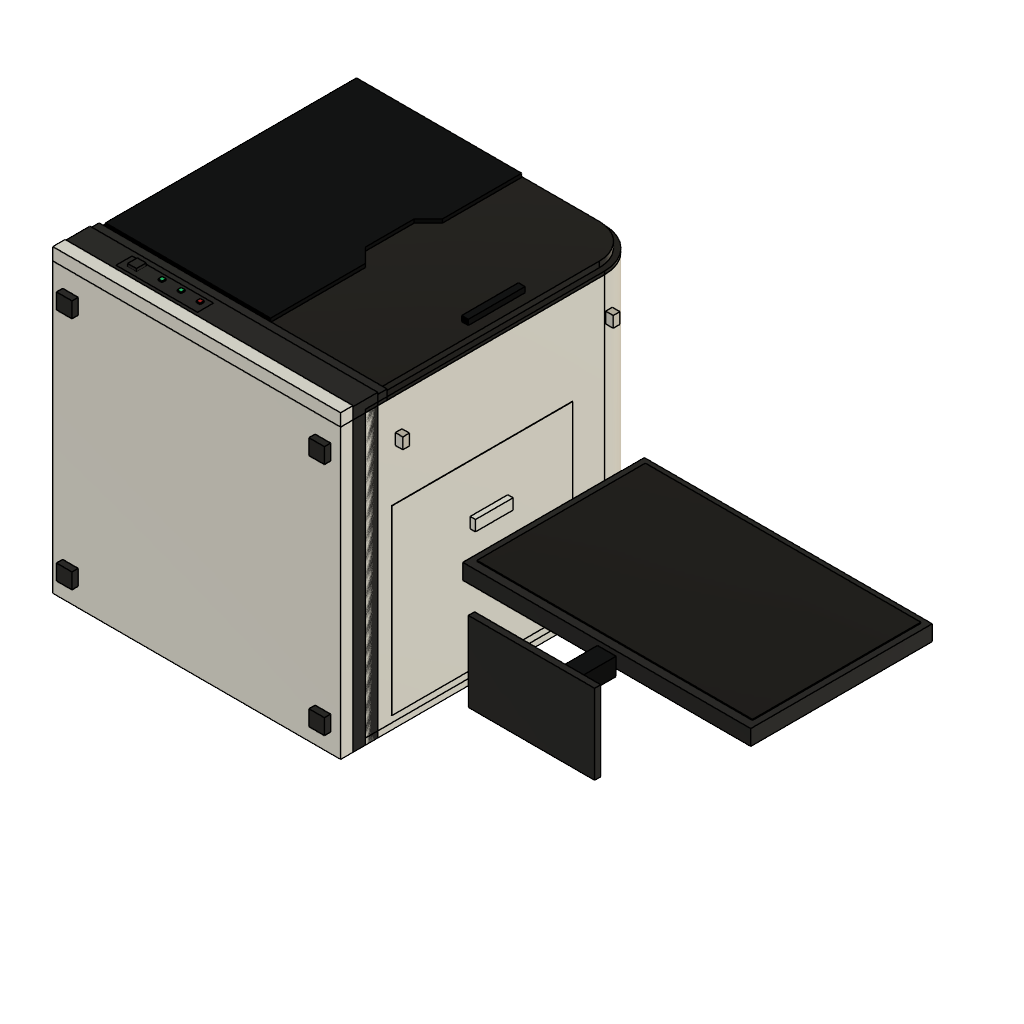
S60-before-branding (Autodesk Fusion 360 design; units mm, degrees)
Autodesk Fusion 360 part; units mm, degrees
(part 1 of 3)
ref_plane "WorkPlane1" through (0, 0, -280) normal (0, 0, 1) x (1, 0, 0) in component "cassette_bays | Three vertical cassette bays | DEPTH PROVISIONAL"
sketch "bay_back profile" plane through (0, 0, -280) normal (0, 0, 1) x (1, 0, 0) in component "cassette_bays | Three vertical cassette bays | DEPTH PROVISIONAL"
  line L0 (142, 117.5) -> (268, 117.5)
  line L1 (268, 117.5) -> (268, 592.5)
  line L2 (268, 592.5) -> (142, 592.5)
  line L3 (142, 592.5) -> (142, 117.5)
extrude "bay_back solid extrusion" add sketch "bay_back profile" along normal blind 9 makes body 1 in component "cassette_bays | Three vertical cassette bays | DEPTH PROVISIONAL"
ref_plane "WorkPlane2" through (0, 0, -275.5) normal (0, 0, 1) x (1, 0, 0) in component "cassette_bays | Three vertical cassette bays | DEPTH PROVISIONAL"
sketch "side_frame profile" plane through (0, 0, -275.5) normal (0, 0, 1) x (1, 0, 0) in component "cassette_bays | Three vertical cassette bays | DEPTH PROVISIONAL"
  line L0 (140, 118) -> (150, 118)
  line L1 (150, 118) -> (150, 592)
  line L2 (150, 592) -> (140, 592)
  line L3 (140, 592) -> (140, 118)
  line L4 (260, 118) -> (270, 118)
  line L5 (270, 118) -> (270, 592)
  line L6 (270, 592) -> (260, 592)
  line L7 (260, 592) -> (260, 118)
extrude "side_frame solid extrusion" add sketch "side_frame profile" along normal blind 108 separate body makes body 2 at (140, 434, -239.5) makes body 3 at (260, 434, -239.5) in component "cassette_bays | Three vertical cassette bays | DEPTH PROVISIONAL"
ref_plane "WorkPlane3" through (0, 0, -275.5) normal (0, 0, 1) x (1, 0, 0) in component "cassette_bays | Three vertical cassette bays | DEPTH PROVISIONAL"
sketch "cross_frame profile" plane through (0, 0, -275.5) normal (0, 0, 1) x (1, 0, 0) in component "cassette_bays | Three vertical cassette bays | DEPTH PROVISIONAL"
  line L0 (140, 116) -> (270, 116)
  line L1 (270, 116) -> (270, 126)
  line L2 (270, 126) -> (140, 126)
  line L3 (140, 126) -> (140, 116)
  line L4 (140, 275) -> (270, 275)
  line L5 (270, 275) -> (270, 285)
  line L6 (270, 285) -> (140, 285)
  line L7 (140, 285) -> (140, 275)
  line L8 (140, 425) -> (270, 425)
  line L9 (270, 425) -> (270, 435)
  line L10 (270, 435) -> (140, 435)
  line L11 (140, 435) -> (140, 425)
  line L12 (140, 584) -> (270, 584)
  line L13 (270, 584) -> (270, 594)
  line L14 (270, 594) -> (140, 594)
  line L15 (140, 594) -> (140, 584)
extrude "cross_frame solid extrusion" add sketch "cross_frame profile" along normal blind 108 separate body makes body 4 at (226.6667, 435, -239.5) makes body 5 at (226.6667, 285, -239.5) makes body 6 at (226.6667, 126, -239.5) makes body 7 at (226.6667, 594, -239.5) in component "cassette_bays | Three vertical cassette bays | DEPTH PROVISIONAL"
ref_plane "WorkPlane4" through (0, 0, -165.5) normal (0, 0, 1) x (1, 0, 0) in component "cassette_bays | Three vertical cassette bays | DEPTH PROVISIONAL"
sketch "seat_led_0 profile" plane through (0, 0, -165.5) normal (0, 0, 1) x (1, 0, 0) in component "cassette_bays | Three vertical cassette bays | DEPTH PROVISIONAL"
  line L0 (144, 264) -> (150, 264)
  line L1 (150, 264) -> (150, 270)
  line L2 (150, 270) -> (144, 270)
  line L3 (144, 270) -> (144, 264)
extrude "seat_led_0 solid extrusion" add sketch "seat_led_0 profile" along normal blind 4 separate body makes body 8 in component "cassette_bays | Three vertical cassette bays | DEPTH PROVISIONAL"
ref_plane "WorkPlane5" through (0, 0, -165.5) normal (0, 0, 1) x (1, 0, 0) in component "cassette_bays | Three vertical cassette bays | DEPTH PROVISIONAL"
sketch "seat_led_1 profile" plane through (0, 0, -165.5) normal (0, 0, 1) x (1, 0, 0) in component "cassette_bays | Three vertical cassette bays | DEPTH PROVISIONAL"
  line L0 (144, 414) -> (150, 414)
  line L1 (150, 414) -> (150, 420)
  line L2 (150, 420) -> (144, 420)
  line L3 (144, 420) -> (144, 414)
extrude "seat_led_1 solid extrusion" add sketch "seat_led_1 profile" along normal blind 4 separate body makes body 9 in component "cassette_bays | Three vertical cassette bays | DEPTH PROVISIONAL"
ref_plane "WorkPlane6" through (0, 0, -165.5) normal (0, 0, 1) x (1, 0, 0) in component "cassette_bays | Three vertical cassette bays | DEPTH PROVISIONAL"
sketch "seat_led_2 profile" plane through (0, 0, -165.5) normal (0, 0, 1) x (1, 0, 0) in component "cassette_bays | Three vertical cassette bays | DEPTH PROVISIONAL"
  line L0 (144, 564) -> (150, 564)
  line L1 (150, 564) -> (150, 570)
  line L2 (150, 570) -> (144, 570)
  line L3 (144, 570) -> (144, 564)
extrude "seat_led_2 solid extrusion" add sketch "seat_led_2 profile" along normal blind 4 separate body makes body 10 in component "cassette_bays | Three vertical cassette bays | DEPTH PROVISIONAL"
ref_plane "WorkPlane1" through (0, 0, -269.5) normal (0, 0, 1) x (1, 0, 0) in component "cassette_0 | Bottom cassette | DEPTH PROVISIONAL"
sketch "rack_base profile" plane through (0, 0, -269.5) normal (0, 0, 1) x (1, 0, 0) in component "cassette_0 | Bottom cassette | DEPTH PROVISIONAL"
  line L0 (165, 139) -> (245, 139)
  line L1 (245, 139) -> (245, 145)
  line L2 (245, 145) -> (165, 145)
  line L3 (165, 145) -> (165, 139)
extrude "rack_base solid extrusion" add sketch "rack_base profile" along normal blind 96 separate body makes body 11 in component "cassette_0 | Bottom cassette | DEPTH PROVISIONAL"
ref_plane "WorkPlane2" through (0, 0, -269.5) normal (0, 0, 1) x (1, 0, 0) in component "cassette_0 | Bottom cassette | DEPTH PROVISIONAL"
sketch "rack_top profile" plane through (0, 0, -269.5) normal (0, 0, 1) x (1, 0, 0) in component "cassette_0 | Bottom cassette | DEPTH PROVISIONAL"
  line L0 (165, 265.5) -> (245, 265.5)
  line L1 (245, 265.5) -> (245, 270.5)
  line L2 (245, 270.5) -> (165, 270.5)
  line L3 (165, 270.5) -> (165, 265.5)
extrude "rack_top solid extrusion" add sketch "rack_top profile" along normal blind 96 separate body makes body 12 in component "cassette_0 | Bottom cassette | DEPTH PROVISIONAL"
ref_plane "WorkPlane3" through (0, 0, -269.5) normal (0, 0, 1) x (1, 0, 0) in component "cassette_0 | Bottom cassette | DEPTH PROVISIONAL"
sketch "outer_guide profile" plane through (0, 0, -269.5) normal (0, 0, 1) x (1, 0, 0) in component "cassette_0 | Bottom cassette | DEPTH PROVISIONAL"
  line L0 (165, 143.5) -> (169, 143.5)
  line L1 (169, 143.5) -> (169, 266.5)
  line L2 (169, 266.5) -> (165, 266.5)
  line L3 (165, 266.5) -> (165, 143.5)
  line L4 (241, 143.5) -> (245, 143.5)
  line L5 (245, 143.5) -> (245, 266.5)
  line L6 (245, 266.5) -> (241, 266.5)
  line L7 (241, 266.5) -> (241, 143.5)
extrude "outer_guide solid extrusion" add sketch "outer_guide profile" along normal blind 96 separate body makes body 13 at (165, 225.5, -237.5) makes body 14 at (241, 225.5, -237.5) in component "cassette_0 | Bottom cassette | DEPTH PROVISIONAL"
ref_plane "WorkPlane4" through (0, 0, -177.5) normal (0, 0, 1) x (1, 0, 0) in component "cassette_0 | Bottom cassette | DEPTH PROVISIONAL"
sketch "rear_rib_PHOTO_ESTIMATE profile" plane through (0, 0, -177.5) normal (0, 0, 1) x (1, 0, 0) in component "cassette_0 | Bottom cassette | DEPTH PROVISIONAL"
  line L0 (168.5, 144) -> (175.5, 144)
  line L1 (175.5, 144) -> (175.5, 266)
  line L2 (175.5, 266) -> (168.5, 266)
  line L3 (168.5, 266) -> (168.5, 144)
  line L4 (201.5, 144) -> (208.5, 144)
  line L5 (208.5, 144) -> (208.5, 266)
  line L6 (208.5, 266) -> (201.5, 266)
  line L7 (201.5, 266) -> (201.5, 144)
  line L8 (234.5, 144) -> (241.5, 144)
  line L9 (241.5, 144) -> (241.5, 266)
  line L10 (241.5, 266) -> (234.5, 266)
  line L11 (234.5, 266) -> (234.5, 144)
extrude "rear_rib_PHOTO_ESTIMATE solid extrusion" add sketch "rear_rib_PHOTO_ESTIMATE profile" along normal blind 4 separate body makes body 15 at (170.8333, 184.6667, -177.5) makes body 16 at (203.8333, 225.3333, -177.5) makes body 17 at (236.8333, 184.6667, -177.5) in component "cassette_0 | Bottom cassette | DEPTH PROVISIONAL"
ref_plane "WorkPlane5" through (0, 0, -234) normal (0, 0, 1) x (1, 0, 0) in component "cassette_0 | Bottom cassette | DEPTH PROVISIONAL"
sketch "magnetic_base profile" plane through (0, 0, -234) normal (0, 0, 1) x (1, 0, 0) in component "cassette_0 | Bottom cassette | DEPTH PROVISIONAL"
  line L0 (191, 136.5) -> (219, 136.5)
  line L1 (219, 136.5) -> (219, 139.5)
  line L2 (219, 139.5) -> (191, 139.5)
  line L3 (191, 139.5) -> (191, 136.5)
extrude "magnetic_base solid extrusion" add sketch "magnetic_base profile" along normal blind 25 separate body makes body 18 in component "cassette_0 | Bottom cassette | DEPTH PROVISIONAL"
ref_plane "WorkPlane6" through (0, 0, -269.5) normal (0, 0, 1) x (1, 0, 0) in component "cassette_0 | Bottom cassette | DEPTH PROVISIONAL"
sketch "center_divider profile" plane through (0, 0, -269.5) normal (0, 0, 1) x (1, 0, 0) in component "cassette_0 | Bottom cassette | DEPTH PROVISIONAL"
  line L0 (203, 144) -> (207, 144)
  line L1 (207, 144) -> (207, 266)
  line L2 (207, 266) -> (203, 266)
  line L3 (203, 266) -> (203, 144)
extrude "center_divider solid extrusion" add sketch "center_divider profile" along normal blind 96 separate body makes body 19 in component "cassette_0 | Bottom cassette | DEPTH PROVISIONAL"
ref_plane "WorkPlane7" through (0, 0, -259.5) normal (0, 0, 1) x (1, 0, 0) in component "cassette_0 | Bottom cassette | DEPTH PROVISIONAL"
sketch "slide_glass profile" plane through (0, 0, -259.5) normal (0, 0, 1) x (1, 0, 0) in component "cassette_0 | Bottom cassette | DEPTH PROVISIONAL"
  line L0 (175, 253.5) -> (201, 253.5)
  line L1 (201, 253.5) -> (201, 254.5)
  line L2 (201, 254.5) -> (175, 254.5)
  line L3 (175, 254.5) -> (175, 253.5)
  line L4 (175, 243) -> (201, 243)
  line L5 (201, 243) -> (201, 244)
  line L6 (201, 244) -> (175, 244)
  line L7 (175, 244) -> (175, 243)
  line L8 (175, 232.5) -> (201, 232.5)
  line L9 (201, 232.5) -> (201, 233.5)
  line L10 (201, 233.5) -> (175, 233.5)
  line L11 (175, 233.5) -> (175, 232.5)
  line L12 (175, 222) -> (201, 222)
  line L13 (201, 222) -> (201, 223)
  line L14 (201, 223) -> (175, 223)
  line L15 (175, 223) -> (175, 222)
  line L16 (175, 211.5) -> (201, 211.5)
  line L17 (201, 211.5) -> (201, 212.5)
  line L18 (201, 212.5) -> (175, 212.5)
  line L19 (175, 212.5) -> (175, 211.5)
  line L20 (175, 201) -> (201, 201)
  line L21 (201, 201) -> (201, 202)
  line L22 (201, 202) -> (175, 202)
  line L23 (175, 202) -> (175, 201)
  line L24 (175, 190.5) -> (201, 190.5)
  line L25 (201, 190.5) -> (201, 191.5)
  line L26 (201, 191.5) -> (175, 191.5)
  line L27 (175, 191.5) -> (175, 190.5)
  line L28 (175, 180) -> (201, 180)
  line L29 (201, 180) -> (201, 181)
  line L30 (201, 181) -> (175, 181)
  line L31 (175, 181) -> (175, 180)
  line L32 (175, 169.5) -> (201, 169.5)
  line L33 (201, 169.5) -> (201, 170.5)
  line L34 (201, 170.5) -> (175, 170.5)
  line L35 (175, 170.5) -> (175, 169.5)
  line L36 (175, 159) -> (201, 159)
  line L37 (201, 159) -> (201, 160)
  line L38 (201, 160) -> (175, 160)
  line L39 (175, 160) -> (175, 159)
  line L40 (209, 253.5) -> (235, 253.5)
  line L41 (235, 253.5) -> (235, 254.5)
  line L42 (235, 254.5) -> (209, 254.5)
  line L43 (209, 254.5) -> (209, 253.5)
  line L44 (209, 243) -> (235, 243)
  line L45 (235, 243) -> (235, 244)
  line L46 (235, 244) -> (209, 244)
  line L47 (209, 244) -> (209, 243)
  line L48 (209, 232.5) -> (235, 232.5)
  line L49 (235, 232.5) -> (235, 233.5)
  line L50 (235, 233.5) -> (209, 233.5)
  line L51 (209, 233.5) -> (209, 232.5)
  line L52 (209, 222) -> (235, 222)
  line L53 (235, 222) -> (235, 223)
  line L54 (235, 223) -> (209, 223)
  line L55 (209, 223) -> (209, 222)
  line L56 (209, 211.5) -> (235, 211.5)
  line L57 (235, 211.5) -> (235, 212.5)
  line L58 (235, 212.5) -> (209, 212.5)
  line L59 (209, 212.5) -> (209, 211.5)
  line L60 (209, 201) -> (235, 201)
  line L61 (235, 201) -> (235, 202)
  line L62 (235, 202) -> (209, 202)
  line L63 (209, 202) -> (209, 201)
  line L64 (209, 190.5) -> (235, 190.5)
  line L65 (235, 190.5) -> (235, 191.5)
  line L66 (235, 191.5) -> (209, 191.5)
  line L67 (209, 191.5) -> (209, 190.5)
  line L68 (209, 180) -> (235, 180)
  line L69 (235, 180) -> (235, 181)
  line L70 (235, 181) -> (209, 181)
  line L71 (209, 181) -> (209, 180)
  line L72 (209, 169.5) -> (235, 169.5)
  line L73 (235, 169.5) -> (235, 170.5)
  line L74 (235, 170.5) -> (209, 170.5)
  line L75 (209, 170.5) -> (209, 169.5)
  line L76 (209, 159) -> (235, 159)
  line L77 (235, 159) -> (235, 160)
  line L78 (235, 160) -> (209, 160)
  line L79 (209, 160) -> (209, 159)
extrude "slide_glass solid extrusion" add sketch "slide_glass profile" along normal blind 76 separate body makes body 20 at (226.3333, 170.5, -234.1667) makes body 21 at (226.3333, 191.5, -234.1667) makes body 22 at (226.3333, 212.5, -234.1667) makes body 23 at (226.3333, 233.5, -234.1667) makes body 24 at (226.3333, 254.5, -234.1667) makes body 25 at (192.3333, 160, -234.1667) makes body 26 at (192.3333, 181, -234.1667) makes body 27 at (192.3333, 202, -234.1667) makes body 28 at (192.3333, 223, -234.1667) makes body 29 at (192.3333, 244, -234.1667) makes body 30 at (192.3333, 233.5, -234.1667) makes body 31 at (192.3333, 212.5, -234.1667) makes body 32 at (192.3333, 191.5, -234.1667) makes body 33 at (192.3333, 170.5, -234.1667) makes body 34 at (192.3333, 254.5, -234.1667) makes body 35 at (226.3333, 244, -234.1667) makes body 36 at (226.3333, 223, -234.1667) makes body 37 at (226.3333, 202, -234.1667) makes body 38 at (226.3333, 181, -234.1667) makes body 39 at (226.3333, 160, -234.1667) in component "cassette_0 | Bottom cassette | DEPTH PROVISIONAL"
ref_plane "WorkPlane8" through (0, 0, -263) normal (0, 0, 1) x (1, 0, 0) in component "cassette_0 | Bottom cassette | DEPTH PROVISIONAL"
sketch "slot_guide profile" plane through (0, 0, -263) normal (0, 0, 1) x (1, 0, 0) in component "cassette_0 | Bottom cassette | DEPTH PROVISIONAL"
  line L0 (173, 252) -> (175, 252)
  line L1 (175, 252) -> (175, 254)
  line L2 (175, 254) -> (173, 254)
  line L3 (173, 254) -> (173, 252)
  line L4 (201, 252) -> (203, 252)
  line L5 (203, 252) -> (203, 254)
  line L6 (203, 254) -> (201, 254)
  line L7 (201, 254) -> (201, 252)
  line L8 (173, 241.5) -> (175, 241.5)
  line L9 (175, 241.5) -> (175, 243.5)
  line L10 (175, 243.5) -> (173, 243.5)
  line L11 (173, 243.5) -> (173, 241.5)
  line L12 (201, 241.5) -> (203, 241.5)
  line L13 (203, 241.5) -> (203, 243.5)
  line L14 (203, 243.5) -> (201, 243.5)
  line L15 (201, 243.5) -> (201, 241.5)
  line L16 (173, 231) -> (175, 231)
  line L17 (175, 231) -> (175, 233)
  line L18 (175, 233) -> (173, 233)
  line L19 (173, 233) -> (173, 231)
  line L20 (201, 231) -> (203, 231)
  line L21 (203, 231) -> (203, 233)
  line L22 (203, 233) -> (201, 233)
  line L23 (201, 233) -> (201, 231)
  line L24 (173, 220.5) -> (175, 220.5)
  line L25 (175, 220.5) -> (175, 222.5)
  line L26 (175, 222.5) -> (173, 222.5)
  line L27 (173, 222.5) -> (173, 220.5)
  line L28 (201, 220.5) -> (203, 220.5)
  line L29 (203, 220.5) -> (203, 222.5)
  line L30 (203, 222.5) -> (201, 222.5)
  line L31 (201, 222.5) -> (201, 220.5)
  line L32 (173, 210) -> (175, 210)
  line L33 (175, 210) -> (175, 212)
  line L34 (175, 212) -> (173, 212)
  line L35 (173, 212) -> (173, 210)
  line L36 (201, 210) -> (203, 210)
  line L37 (203, 210) -> (203, 212)
  line L38 (203, 212) -> (201, 212)
  line L39 (201, 212) -> (201, 210)
  line L40 (173, 199.5) -> (175, 199.5)
  line L41 (175, 199.5) -> (175, 201.5)
  line L42 (175, 201.5) -> (173, 201.5)
  line L43 (173, 201.5) -> (173, 199.5)
  line L44 (201, 199.5) -> (203, 199.5)
  line L45 (203, 199.5) -> (203, 201.5)
  line L46 (203, 201.5) -> (201, 201.5)
  line L47 (201, 201.5) -> (201, 199.5)
  line L48 (173, 189) -> (175, 189)
  line L49 (175, 189) -> (175, 191)
  line L50 (175, 191) -> (173, 191)
  line L51 (173, 191) -> (173, 189)
  line L52 (201, 189) -> (203, 189)
  line L53 (203, 189) -> (203, 191)
  line L54 (203, 191) -> (201, 191)
  line L55 (201, 191) -> (201, 189)
  line L56 (173, 178.5) -> (175, 178.5)
  line L57 (175, 178.5) -> (175, 180.5)
  line L58 (175, 180.5) -> (173, 180.5)
  line L59 (173, 180.5) -> (173, 178.5)
  line L60 (201, 178.5) -> (203, 178.5)
  line L61 (203, 178.5) -> (203, 180.5)
  line L62 (203, 180.5) -> (201, 180.5)
  line L63 (201, 180.5) -> (201, 178.5)
  line L64 (173, 168) -> (175, 168)
  line L65 (175, 168) -> (175, 170)
  line L66 (175, 170) -> (173, 170)
  line L67 (173, 170) -> (173, 168)
  line L68 (201, 168) -> (203, 168)
  line L69 (203, 168) -> (203, 170)
  line L70 (203, 170) -> (201, 170)
  line L71 (201, 170) -> (201, 168)
  line L72 (173, 157.5) -> (175, 157.5)
  line L73 (175, 157.5) -> (175, 159.5)
  line L74 (175, 159.5) -> (173, 159.5)
  line L75 (173, 159.5) -> (173, 157.5)
  line L76 (201, 157.5) -> (203, 157.5)
  line L77 (203, 157.5) -> (203, 159.5)
  line L78 (203, 159.5) -> (201, 159.5)
  line L79 (201, 159.5) -> (201, 157.5)
  line L80 (207, 252) -> (209, 252)
  line L81 (209, 252) -> (209, 254)
  line L82 (209, 254) -> (207, 254)
  line L83 (207, 254) -> (207, 252)
  line L84 (235, 252) -> (237, 252)
  line L85 (237, 252) -> (237, 254)
  line L86 (237, 254) -> (235, 254)
  line L87 (235, 254) -> (235, 252)
  line L88 (207, 241.5) -> (209, 241.5)
  line L89 (209, 241.5) -> (209, 243.5)
  line L90 (209, 243.5) -> (207, 243.5)
  line L91 (207, 243.5) -> (207, 241.5)
  line L92 (235, 241.5) -> (237, 241.5)
  line L93 (237, 241.5) -> (237, 243.5)
  line L94 (237, 243.5) -> (235, 243.5)
  line L95 (235, 243.5) -> (235, 241.5)
  line L96 (207, 231) -> (209, 231)
  line L97 (209, 231) -> (209, 233)
  line L98 (209, 233) -> (207, 233)
  line L99 (207, 233) -> (207, 231)
  line L100 (235, 231) -> (237, 231)
  line L101 (237, 231) -> (237, 233)
  line L102 (237, 233) -> (235, 233)
  line L103 (235, 233) -> (235, 231)
  line L104 (207, 220.5) -> (209, 220.5)
  line L105 (209, 220.5) -> (209, 222.5)
  line L106 (209, 222.5) -> (207, 222.5)
  line L107 (207, 222.5) -> (207, 220.5)
  line L108 (235, 220.5) -> (237, 220.5)
  line L109 (237, 220.5) -> (237, 222.5)
  line L110 (237, 222.5) -> (235, 222.5)
  line L111 (235, 222.5) -> (235, 220.5)
  line L112 (207, 210) -> (209, 210)
  line L113 (209, 210) -> (209, 212)
  line L114 (209, 212) -> (207, 212)
  line L115 (207, 212) -> (207, 210)
  line L116 (235, 210) -> (237, 210)
  line L117 (237, 210) -> (237, 212)
  line L118 (237, 212) -> (235, 212)
  line L119 (235, 212) -> (235, 210)
  line L120 (207, 199.5) -> (209, 199.5)
  line L121 (209, 199.5) -> (209, 201.5)
  line L122 (209, 201.5) -> (207, 201.5)
  line L123 (207, 201.5) -> (207, 199.5)
  line L124 (235, 199.5) -> (237, 199.5)
  line L125 (237, 199.5) -> (237, 201.5)
  line L126 (237, 201.5) -> (235, 201.5)
  line L127 (235, 201.5) -> (235, 199.5)
  line L128 (207, 189) -> (209, 189)
  line L129 (209, 189) -> (209, 191)
  line L130 (209, 191) -> (207, 191)
  line L131 (207, 191) -> (207, 189)
  line L132 (235, 189) -> (237, 189)
  line L133 (237, 189) -> (237, 191)
  line L134 (237, 191) -> (235, 191)
  line L135 (235, 191) -> (235, 189)
  line L136 (207, 178.5) -> (209, 178.5)
  line L137 (209, 178.5) -> (209, 180.5)
  line L138 (209, 180.5) -> (207, 180.5)
  line L139 (207, 180.5) -> (207, 178.5)
  line L140 (235, 178.5) -> (237, 178.5)
  line L141 (237, 178.5) -> (237, 180.5)
  line L142 (237, 180.5) -> (235, 180.5)
  line L143 (235, 180.5) -> (235, 178.5)
  line L144 (207, 168) -> (209, 168)
  line L145 (209, 168) -> (209, 170)
  line L146 (209, 170) -> (207, 170)
  line L147 (207, 170) -> (207, 168)
  line L148 (235, 168) -> (237, 168)
  line L149 (237, 168) -> (237, 170)
  line L150 (237, 170) -> (235, 170)
  line L151 (235, 170) -> (235, 168)
  line L152 (207, 157.5) -> (209, 157.5)
  line L153 (209, 157.5) -> (209, 159.5)
  line L154 (209, 159.5) -> (207, 159.5)
  line L155 (207, 159.5) -> (207, 157.5)
  line L156 (235, 157.5) -> (237, 157.5)
  line L157 (237, 157.5) -> (237, 159.5)
  line L158 (237, 159.5) -> (235, 159.5)
  line L159 (235, 159.5) -> (235, 157.5)
extrude "slot_guide solid extrusion" add sketch "slot_guide profile" along normal blind 83 separate body makes body 40 at (207, 158.8333, -207.6667) makes body 41 at (207, 169.3333, -207.6667) makes body 42 at (207, 179.8333, -207.6667) makes body 43 at (209, 189.6667, -207.6667) makes body 44 at (207, 200.8333, -207.6667) makes body 45 at (207, 211.3333, -207.6667) makes body 46 at (207, 221.8333, -207.6667) makes body 47 at (207, 232.3333, -207.6667) makes body 48 at (209, 242.1667, -207.6667) makes body 49 at (207, 253.3333, -207.6667) makes body 50 at (201, 158.8333, -207.6667) makes body 51 at (201, 169.3333, -207.6667) makes body 52 at (201, 179.8333, -207.6667) makes body 53 at (203, 189.6667, -207.6667) makes body 54 at (201, 200.8333, -207.6667) makes body 55 at (201, 211.3333, -207.6667) makes body 56 at (201, 221.8333, -207.6667) makes body 57 at (201, 232.3333, -207.6667) makes body 58 at (203, 242.1667, -207.6667) makes body 59 at (201, 253.3333, -207.6667) makes body 60 at (175, 242.1667, -207.6667) makes body 61 at (173, 232.3333, -207.6667) makes body 62 at (173, 221.8333, -207.6667) makes body 63 at (173, 211.3333, -207.6667) makes body 64 at (173, 200.8333, -207.6667) makes body 65 at (175, 189.6667, -207.6667) makes body 66 at (173, 179.8333, -207.6667) makes body 67 at (173, 169.3333, -207.6667) makes body 68 at (173, 158.8333, -207.6667) makes body 69 at (173, 253.3333, -207.6667) makes body 70 at (235, 253.3333, -207.6667) makes body 71 at (237, 242.1667, -207.6667) makes body 72 at (235, 232.3333, -207.6667) makes body 73 at (235, 221.8333, -207.6667) makes body 74 at (235, 211.3333, -207.6667) makes body 75 at (235, 200.8333, -207.6667) makes body 76 at (237, 189.6667, -207.6667) makes body 77 at (235, 179.8333, -207.6667) makes body 78 at (235, 169.3333, -207.6667) makes body 79 at (235, 158.8333, -207.6667) in component "cassette_0 | Bottom cassette | DEPTH PROVISIONAL"
ref_plane "WorkPlane1" through (0, 0, -269.5) normal (0, 0, 1) x (1, 0, 0) in component "cassette_1 | Middle cassette | DEPTH PROVISIONAL"
sketch "rack_base profile (2)" plane through (0, 0, -269.5) normal (0, 0, 1) x (1, 0, 0) in component "cassette_1 | Middle cassette | DEPTH PROVISIONAL"
  line L0 (165, 289) -> (245, 289)
  line L1 (245, 289) -> (245, 295)
  line L2 (245, 295) -> (165, 295)
  line L3 (165, 295) -> (165, 289)
extrude "rack_base solid extrusion'" add sketch "rack_base profile (2)" along normal blind 96 separate body makes body 80 in component "cassette_1 | Middle cassette | DEPTH PROVISIONAL"
ref_plane "WorkPlane2" through (0, 0, -269.5) normal (0, 0, 1) x (1, 0, 0) in component "cassette_1 | Middle cassette | DEPTH PROVISIONAL"
sketch "rack_top profile (2)" plane through (0, 0, -269.5) normal (0, 0, 1) x (1, 0, 0) in component "cassette_1 | Middle cassette | DEPTH PROVISIONAL"
  line L0 (165, 415.5) -> (245, 415.5)
  line L1 (245, 415.5) -> (245, 420.5)
  line L2 (245, 420.5) -> (165, 420.5)
  line L3 (165, 420.5) -> (165, 415.5)
extrude "rack_top solid extrusion'" add sketch "rack_top profile (2)" along normal blind 96 separate body makes body 81 in component "cassette_1 | Middle cassette | DEPTH PROVISIONAL"
ref_plane "WorkPlane3" through (0, 0, -269.5) normal (0, 0, 1) x (1, 0, 0) in component "cassette_1 | Middle cassette | DEPTH PROVISIONAL"
sketch "outer_guide profile (2)" plane through (0, 0, -269.5) normal (0, 0, 1) x (1, 0, 0) in component "cassette_1 | Middle cassette | DEPTH PROVISIONAL"
  line L0 (165, 293.5) -> (169, 293.5)
  line L1 (169, 293.5) -> (169, 416.5)
  line L2 (169, 416.5) -> (165, 416.5)
  line L3 (165, 416.5) -> (165, 293.5)
  line L4 (241, 293.5) -> (245, 293.5)
  line L5 (245, 293.5) -> (245, 416.5)
  line L6 (245, 416.5) -> (241, 416.5)
  line L7 (241, 416.5) -> (241, 293.5)
extrude "outer_guide solid extrusion'" add sketch "outer_guide profile (2)" along normal blind 96 separate body makes body 82 at (165, 375.5, -237.5) makes body 83 at (241, 375.5, -237.5) in component "cassette_1 | Middle cassette | DEPTH PROVISIONAL"
ref_plane "WorkPlane4" through (0, 0, -177.5) normal (0, 0, 1) x (1, 0, 0) in component "cassette_1 | Middle cassette | DEPTH PROVISIONAL"
sketch "rear_rib_PHOTO_ESTIMATE profile (2)" plane through (0, 0, -177.5) normal (0, 0, 1) x (1, 0, 0) in component "cassette_1 | Middle cassette | DEPTH PROVISIONAL"
  line L0 (168.5, 294) -> (175.5, 294)
  line L1 (175.5, 294) -> (175.5, 416)
  line L2 (175.5, 416) -> (168.5, 416)
  line L3 (168.5, 416) -> (168.5, 294)
  line L4 (201.5, 294) -> (208.5, 294)
  line L5 (208.5, 294) -> (208.5, 416)
  line L6 (208.5, 416) -> (201.5, 416)
  line L7 (201.5, 416) -> (201.5, 294)
  line L8 (234.5, 294) -> (241.5, 294)
  line L9 (241.5, 294) -> (241.5, 416)
  line L10 (241.5, 416) -> (234.5, 416)
  line L11 (234.5, 416) -> (234.5, 294)
extrude "rear_rib_PHOTO_ESTIMATE solid extrusion'" add sketch "rear_rib_PHOTO_ESTIMATE profile (2)" along normal blind 4 separate body makes body 84 at (170.8333, 375.3333, -177.5) makes body 85 at (203.8333, 375.3333, -177.5) makes body 86 at (236.8333, 375.3333, -177.5) in component "cassette_1 | Middle cassette | DEPTH PROVISIONAL"
ref_plane "WorkPlane5" through (0, 0, -234) normal (0, 0, 1) x (1, 0, 0) in component "cassette_1 | Middle cassette | DEPTH PROVISIONAL"
sketch "magnetic_base profile (2)" plane through (0, 0, -234) normal (0, 0, 1) x (1, 0, 0) in component "cassette_1 | Middle cassette | DEPTH PROVISIONAL"
  line L0 (191, 286.5) -> (219, 286.5)
  line L1 (219, 286.5) -> (219, 289.5)
  line L2 (219, 289.5) -> (191, 289.5)
  line L3 (191, 289.5) -> (191, 286.5)
extrude "magnetic_base solid extrusion'" add sketch "magnetic_base profile (2)" along normal blind 25 separate body makes body 87 in component "cassette_1 | Middle cassette | DEPTH PROVISIONAL"
ref_plane "WorkPlane6" through (0, 0, -269.5) normal (0, 0, 1) x (1, 0, 0) in component "cassette_1 | Middle cassette | DEPTH PROVISIONAL"
sketch "center_divider profile (2)" plane through (0, 0, -269.5) normal (0, 0, 1) x (1, 0, 0) in component "cassette_1 | Middle cassette | DEPTH PROVISIONAL"
  line L0 (203, 294) -> (207, 294)
  line L1 (207, 294) -> (207, 416)
  line L2 (207, 416) -> (203, 416)
  line L3 (203, 416) -> (203, 294)
extrude "center_divider solid extrusion'" add sketch "center_divider profile (2)" along normal blind 96 separate body makes body 88 in component "cassette_1 | Middle cassette | DEPTH PROVISIONAL"
ref_plane "WorkPlane7" through (0, 0, -259.5) normal (0, 0, 1) x (1, 0, 0) in component "cassette_1 | Middle cassette | DEPTH PROVISIONAL"
sketch "slide_glass profile (2)" plane through (0, 0, -259.5) normal (0, 0, 1) x (1, 0, 0) in component "cassette_1 | Middle cassette | DEPTH PROVISIONAL"
  line L0 (175, 403.5) -> (201, 403.5)
  line L1 (201, 403.5) -> (201, 404.5)
  line L2 (201, 404.5) -> (175, 404.5)
  line L3 (175, 404.5) -> (175, 403.5)
  line L4 (175, 393) -> (201, 393)
  line L5 (201, 393) -> (201, 394)
  line L6 (201, 394) -> (175, 394)
  line L7 (175, 394) -> (175, 393)
  line L8 (175, 382.5) -> (201, 382.5)
  line L9 (201, 382.5) -> (201, 383.5)
  line L10 (201, 383.5) -> (175, 383.5)
  line L11 (175, 383.5) -> (175, 382.5)
  line L12 (175, 372) -> (201, 372)
  line L13 (201, 372) -> (201, 373)
  line L14 (201, 373) -> (175, 373)
  line L15 (175, 373) -> (175, 372)
  line L16 (175, 361.5) -> (201, 361.5)
  line L17 (201, 361.5) -> (201, 362.5)
  line L18 (201, 362.5) -> (175, 362.5)
  line L19 (175, 362.5) -> (175, 361.5)
  line L20 (175, 351) -> (201, 351)
  line L21 (201, 351) -> (201, 352)
  line L22 (201, 352) -> (175, 352)
  line L23 (175, 352) -> (175, 351)
  line L24 (175, 340.5) -> (201, 340.5)
  line L25 (201, 340.5) -> (201, 341.5)
  line L26 (201, 341.5) -> (175, 341.5)
  line L27 (175, 341.5) -> (175, 340.5)
  line L28 (175, 330) -> (201, 330)
  line L29 (201, 330) -> (201, 331)
  line L30 (201, 331) -> (175, 331)
  line L31 (175, 331) -> (175, 330)
  line L32 (175, 319.5) -> (201, 319.5)
  line L33 (201, 319.5) -> (201, 320.5)
  line L34 (201, 320.5) -> (175, 320.5)
  line L35 (175, 320.5) -> (175, 319.5)
  line L36 (175, 309) -> (201, 309)
  line L37 (201, 309) -> (201, 310)
  line L38 (201, 310) -> (175, 310)
  line L39 (175, 310) -> (175, 309)
  line L40 (209, 403.5) -> (235, 403.5)
  line L41 (235, 403.5) -> (235, 404.5)
  line L42 (235, 404.5) -> (209, 404.5)
  line L43 (209, 404.5) -> (209, 403.5)
  line L44 (209, 393) -> (235, 393)
  line L45 (235, 393) -> (235, 394)
  line L46 (235, 394) -> (209, 394)
  line L47 (209, 394) -> (209, 393)
  line L48 (209, 382.5) -> (235, 382.5)
  line L49 (235, 382.5) -> (235, 383.5)
  line L50 (235, 383.5) -> (209, 383.5)
  line L51 (209, 383.5) -> (209, 382.5)
  line L52 (209, 372) -> (235, 372)
  line L53 (235, 372) -> (235, 373)
  line L54 (235, 373) -> (209, 373)
  line L55 (209, 373) -> (209, 372)
  line L56 (209, 361.5) -> (235, 361.5)
  line L57 (235, 361.5) -> (235, 362.5)
  line L58 (235, 362.5) -> (209, 362.5)
  line L59 (209, 362.5) -> (209, 361.5)
  line L60 (209, 351) -> (235, 351)
  line L61 (235, 351) -> (235, 352)
  line L62 (235, 352) -> (209, 352)
  line L63 (209, 352) -> (209, 351)
  line L64 (209, 340.5) -> (235, 340.5)
  line L65 (235, 340.5) -> (235, 341.5)
  line L66 (235, 341.5) -> (209, 341.5)
  line L67 (209, 341.5) -> (209, 340.5)
  line L68 (209, 330) -> (235, 330)
  line L69 (235, 330) -> (235, 331)
  line L70 (235, 331) -> (209, 331)
  line L71 (209, 331) -> (209, 330)
  line L72 (209, 319.5) -> (235, 319.5)
  line L73 (235, 319.5) -> (235, 320.5)
  line L74 (235, 320.5) -> (209, 320.5)
  line L75 (209, 320.5) -> (209, 319.5)
  line L76 (209, 309) -> (235, 309)
  line L77 (235, 309) -> (235, 310)
  line L78 (235, 310) -> (209, 310)
  line L79 (209, 310) -> (209, 309)
extrude "slide_glass solid extrusion'" add sketch "slide_glass profile (2)" along normal blind 76 separate body makes body 89 at (226.3333, 320.5, -234.1667) makes body 90 at (226.3333, 341.5, -234.1667) makes body 91 at (226.3333, 362.5, -234.1667) makes body 92 at (226.3333, 383.5, -234.1667) makes body 93 at (226.3333, 404.5, -234.1667) makes body 94 at (192.3333, 310, -234.1667) makes body 95 at (192.3333, 331, -234.1667) makes body 96 at (192.3333, 352, -234.1667) makes body 97 at (192.3333, 373, -234.1667) makes body 98 at (192.3333, 394, -234.1667) makes body 99 at (192.3333, 383.5, -234.1667) makes body 100 at (192.3333, 362.5, -234.1667) makes body 101 at (192.3333, 341.5, -234.1667) makes body 102 at (192.3333, 320.5, -234.1667) makes body 103 at (192.3333, 404.5, -234.1667) makes body 104 at (226.3333, 394, -234.1667) makes body 105 at (226.3333, 373, -234.1667) makes body 106 at (226.3333, 352, -234.1667) makes body 107 at (226.3333, 331, -234.1667) makes body 108 at (226.3333, 310, -234.1667) in component "cassette_1 | Middle cassette | DEPTH PROVISIONAL"
ref_plane "WorkPlane8" through (0, 0, -263) normal (0, 0, 1) x (1, 0, 0) in component "cassette_1 | Middle cassette | DEPTH PROVISIONAL"
sketch "slot_guide profile (2)" plane through (0, 0, -263) normal (0, 0, 1) x (1, 0, 0) in component "cassette_1 | Middle cassette | DEPTH PROVISIONAL"
  line L0 (173, 402) -> (175, 402)
  line L1 (175, 402) -> (175, 404)
  line L2 (175, 404) -> (173, 404)
  line L3 (173, 404) -> (173, 402)
  line L4 (201, 402) -> (203, 402)
  line L5 (203, 402) -> (203, 404)
  line L6 (203, 404) -> (201, 404)
  line L7 (201, 404) -> (201, 402)
  line L8 (173, 391.5) -> (175, 391.5)
  line L9 (175, 391.5) -> (175, 393.5)
  line L10 (175, 393.5) -> (173, 393.5)
  line L11 (173, 393.5) -> (173, 391.5)
  line L12 (201, 391.5) -> (203, 391.5)
  line L13 (203, 391.5) -> (203, 393.5)
  line L14 (203, 393.5) -> (201, 393.5)
  line L15 (201, 393.5) -> (201, 391.5)
  line L16 (173, 381) -> (175, 381)
  line L17 (175, 381) -> (175, 383)
  line L18 (175, 383) -> (173, 383)
  line L19 (173, 383) -> (173, 381)
  line L20 (201, 381) -> (203, 381)
  line L21 (203, 381) -> (203, 383)
  line L22 (203, 383) -> (201, 383)
  line L23 (201, 383) -> (201, 381)
  line L24 (173, 370.5) -> (175, 370.5)
  line L25 (175, 370.5) -> (175, 372.5)
  line L26 (175, 372.5) -> (173, 372.5)
  line L27 (173, 372.5) -> (173, 370.5)
  line L28 (201, 370.5) -> (203, 370.5)
  line L29 (203, 370.5) -> (203, 372.5)
  line L30 (203, 372.5) -> (201, 372.5)
  line L31 (201, 372.5) -> (201, 370.5)
  line L32 (173, 360) -> (175, 360)
  line L33 (175, 360) -> (175, 362)
  line L34 (175, 362) -> (173, 362)
  line L35 (173, 362) -> (173, 360)
  line L36 (201, 360) -> (203, 360)
  line L37 (203, 360) -> (203, 362)
  line L38 (203, 362) -> (201, 362)
  line L39 (201, 362) -> (201, 360)
  line L40 (173, 349.5) -> (175, 349.5)
  line L41 (175, 349.5) -> (175, 351.5)
  line L42 (175, 351.5) -> (173, 351.5)
  line L43 (173, 351.5) -> (173, 349.5)
  line L44 (201, 349.5) -> (203, 349.5)
  line L45 (203, 349.5) -> (203, 351.5)
  line L46 (203, 351.5) -> (201, 351.5)
  line L47 (201, 351.5) -> (201, 349.5)
  line L48 (173, 339) -> (175, 339)
  line L49 (175, 339) -> (175, 341)
  line L50 (175, 341) -> (173, 341)
  line L51 (173, 341) -> (173, 339)
  line L52 (201, 339) -> (203, 339)
  line L53 (203, 339) -> (203, 341)
  line L54 (203, 341) -> (201, 341)
  line L55 (201, 341) -> (201, 339)
  line L56 (173, 328.5) -> (175, 328.5)
  line L57 (175, 328.5) -> (175, 330.5)
  line L58 (175, 330.5) -> (173, 330.5)
  line L59 (173, 330.5) -> (173, 328.5)
  line L60 (201, 328.5) -> (203, 328.5)
  line L61 (203, 328.5) -> (203, 330.5)
  line L62 (203, 330.5) -> (201, 330.5)
  line L63 (201, 330.5) -> (201, 328.5)
  line L64 (173, 318) -> (175, 318)
  line L65 (175, 318) -> (175, 320)
  line L66 (175, 320) -> (173, 320)
  line L67 (173, 320) -> (173, 318)
  line L68 (201, 318) -> (203, 318)
  line L69 (203, 318) -> (203, 320)
  line L70 (203, 320) -> (201, 320)
  line L71 (201, 320) -> (201, 318)
  line L72 (173, 307.5) -> (175, 307.5)
  line L73 (175, 307.5) -> (175, 309.5)
  line L74 (175, 309.5) -> (173, 309.5)
  line L75 (173, 309.5) -> (173, 307.5)
  line L76 (201, 307.5) -> (203, 307.5)
  line L77 (203, 307.5) -> (203, 309.5)
  line L78 (203, 309.5) -> (201, 309.5)
  line L79 (201, 309.5) -> (201, 307.5)
  line L80 (207, 402) -> (209, 402)
  line L81 (209, 402) -> (209, 404)
  line L82 (209, 404) -> (207, 404)
  line L83 (207, 404) -> (207, 402)
  line L84 (235, 402) -> (237, 402)
  line L85 (237, 402) -> (237, 404)
  line L86 (237, 404) -> (235, 404)
  line L87 (235, 404) -> (235, 402)
  line L88 (207, 391.5) -> (209, 391.5)
  line L89 (209, 391.5) -> (209, 393.5)
  line L90 (209, 393.5) -> (207, 393.5)
  line L91 (207, 393.5) -> (207, 391.5)
  line L92 (235, 391.5) -> (237, 391.5)
  line L93 (237, 391.5) -> (237, 393.5)
  line L94 (237, 393.5) -> (235, 393.5)
  line L95 (235, 393.5) -> (235, 391.5)
  line L96 (207, 381) -> (209, 381)
  line L97 (209, 381) -> (209, 383)
  line L98 (209, 383) -> (207, 383)
  line L99 (207, 383) -> (207, 381)
  line L100 (235, 381) -> (237, 381)
  line L101 (237, 381) -> (237, 383)
  line L102 (237, 383) -> (235, 383)
  line L103 (235, 383) -> (235, 381)
  line L104 (207, 370.5) -> (209, 370.5)
  line L105 (209, 370.5) -> (209, 372.5)
  line L106 (209, 372.5) -> (207, 372.5)
  line L107 (207, 372.5) -> (207, 370.5)
  line L108 (235, 370.5) -> (237, 370.5)
  line L109 (237, 370.5) -> (237, 372.5)
  line L110 (237, 372.5) -> (235, 372.5)
  line L111 (235, 372.5) -> (235, 370.5)
  line L112 (207, 360) -> (209, 360)
  line L113 (209, 360) -> (209, 362)
  line L114 (209, 362) -> (207, 362)
  line L115 (207, 362) -> (207, 360)
  line L116 (235, 360) -> (237, 360)
  line L117 (237, 360) -> (237, 362)
  line L118 (237, 362) -> (235, 362)
  line L119 (235, 362) -> (235, 360)
  line L120 (207, 349.5) -> (209, 349.5)
  line L121 (209, 349.5) -> (209, 351.5)
  line L122 (209, 351.5) -> (207, 351.5)
  line L123 (207, 351.5) -> (207, 349.5)
  line L124 (235, 349.5) -> (237, 349.5)
  line L125 (237, 349.5) -> (237, 351.5)
  line L126 (237, 351.5) -> (235, 351.5)
  line L127 (235, 351.5) -> (235, 349.5)
  line L128 (207, 339) -> (209, 339)
  line L129 (209, 339) -> (209, 341)
  line L130 (209, 341) -> (207, 341)
  line L131 (207, 341) -> (207, 339)
  line L132 (235, 339) -> (237, 339)
  line L133 (237, 339) -> (237, 341)
  line L134 (237, 341) -> (235, 341)
  line L135 (235, 341) -> (235, 339)
  line L136 (207, 328.5) -> (209, 328.5)
  line L137 (209, 328.5) -> (209, 330.5)
  line L138 (209, 330.5) -> (207, 330.5)
  line L139 (207, 330.5) -> (207, 328.5)
  line L140 (235, 328.5) -> (237, 328.5)
  line L141 (237, 328.5) -> (237, 330.5)
  line L142 (237, 330.5) -> (235, 330.5)
  line L143 (235, 330.5) -> (235, 328.5)
  line L144 (207, 318) -> (209, 318)
  line L145 (209, 318) -> (209, 320)
  line L146 (209, 320) -> (207, 320)
  line L147 (207, 320) -> (207, 318)
  line L148 (235, 318) -> (237, 318)
  line L149 (237, 318) -> (237, 320)
  line L150 (237, 320) -> (235, 320)
  line L151 (235, 320) -> (235, 318)
  line L152 (207, 307.5) -> (209, 307.5)
  line L153 (209, 307.5) -> (209, 309.5)
  line L154 (209, 309.5) -> (207, 309.5)
  line L155 (207, 309.5) -> (207, 307.5)
  line L156 (235, 307.5) -> (237, 307.5)
  line L157 (237, 307.5) -> (237, 309.5)
  line L158 (237, 309.5) -> (235, 309.5)
  line L159 (235, 309.5) -> (235, 307.5)
extrude "slot_guide solid extrusion'" add sketch "slot_guide profile (2)" along normal blind 83 separate body makes body 109 at (207, 308.8333, -207.6667) makes body 110 at (207, 319.3333, -207.6667) makes body 111 at (207, 329.8333, -207.6667) makes body 112 at (207, 340.3333, -207.6667) makes body 113 at (207, 350.8333, -207.6667) makes body 114 at (207, 361.3333, -207.6667) makes body 115 at (207, 371.8333, -207.6667) makes body 116 at (207, 382.3333, -207.6667) makes body 117 at (207, 392.8333, -207.6667) makes body 118 at (207, 403.3333, -207.6667) makes body 119 at (201, 308.8333, -207.6667) makes body 120 at (201, 319.3333, -207.6667) makes body 121 at (201, 329.8333, -207.6667) makes body 122 at (201, 340.3333, -207.6667) makes body 123 at (201, 350.8333, -207.6667) makes body 124 at (201, 361.3333, -207.6667) makes body 125 at (201, 371.8333, -207.6667) makes body 126 at (201, 382.3333, -207.6667) makes body 127 at (201, 392.8333, -207.6667) makes body 128 at (201, 403.3333, -207.6667) makes body 129 at (173, 392.8333, -207.6667) makes body 130 at (173, 382.3333, -207.6667) makes body 131 at (173, 371.8333, -207.6667) makes body 132 at (173, 361.3333, -207.6667) makes body 133 at (173, 350.8333, -207.6667) makes body 134 at (173, 340.3333, -207.6667) makes body 135 at (173, 329.8333, -207.6667) makes body 136 at (173, 319.3333, -207.6667) makes body 137 at (173, 308.8333, -207.6667) makes body 138 at (173, 403.3333, -207.6667) makes body 139 at (235, 403.3333, -207.6667) makes body 140 at (235, 392.8333, -207.6667) makes body 141 at (235, 382.3333, -207.6667) makes body 142 at (235, 371.8333, -207.6667) makes body 143 at (235, 361.3333, -207.6667) makes body 144 at (235, 350.8333, -207.6667) makes body 145 at (235, 340.3333, -207.6667) makes body 146 at (235, 329.8333, -207.6667) makes body 147 at (235, 319.3333, -207.6667) makes body 148 at (235, 308.8333, -207.6667) in component "cassette_1 | Middle cassette | DEPTH PROVISIONAL"
ref_plane "WorkPlane1" through (0, 0, -269.5) normal (0, 0, 1) x (1, 0, 0) in component "cassette_2 | Top cassette | DEPTH PROVISIONAL"
sketch "rack_base profile (3)" plane through (0, 0, -269.5) normal (0, 0, 1) x (1, 0, 0) in component "cassette_2 | Top cassette | DEPTH PROVISIONAL"
  line L0 (165, 439) -> (245, 439)
  line L1 (245, 439) -> (245, 445)
  line L2 (245, 445) -> (165, 445)
  line L3 (165, 445) -> (165, 439)
extrude "rack_base solid extrusion''" add sketch "rack_base profile (3)" along normal blind 96 separate body makes body 149 in component "cassette_2 | Top cassette | DEPTH PROVISIONAL"
ref_plane "WorkPlane2" through (0, 0, -269.5) normal (0, 0, 1) x (1, 0, 0) in component "cassette_2 | Top cassette | DEPTH PROVISIONAL"
sketch "rack_top profile (3)" plane through (0, 0, -269.5) normal (0, 0, 1) x (1, 0, 0) in component "cassette_2 | Top cassette | DEPTH PROVISIONAL"
  line L0 (165, 565.5) -> (245, 565.5)
  line L1 (245, 565.5) -> (245, 570.5)
  line L2 (245, 570.5) -> (165, 570.5)
  line L3 (165, 570.5) -> (165, 565.5)
extrude "rack_top solid extrusion''" add sketch "rack_top profile (3)" along normal blind 96 separate body makes body 150 in component "cassette_2 | Top cassette | DEPTH PROVISIONAL"
ref_plane "WorkPlane3" through (0, 0, -269.5) normal (0, 0, 1) x (1, 0, 0) in component "cassette_2 | Top cassette | DEPTH PROVISIONAL"
sketch "outer_guide profile (3)" plane through (0, 0, -269.5) normal (0, 0, 1) x (1, 0, 0) in component "cassette_2 | Top cassette | DEPTH PROVISIONAL"
  line L0 (165, 443.5) -> (169, 443.5)
  line L1 (169, 443.5) -> (169, 566.5)
  line L2 (169, 566.5) -> (165, 566.5)
  line L3 (165, 566.5) -> (165, 443.5)
  line L4 (241, 443.5) -> (245, 443.5)
  line L5 (245, 443.5) -> (245, 566.5)
  line L6 (245, 566.5) -> (241, 566.5)
  line L7 (241, 566.5) -> (241, 443.5)
extrude "outer_guide solid extrusion''" add sketch "outer_guide profile (3)" along normal blind 96 separate body makes body 151 at (165, 525.5, -237.5) makes body 152 at (241, 525.5, -237.5) in component "cassette_2 | Top cassette | DEPTH PROVISIONAL"
ref_plane "WorkPlane4" through (0, 0, -177.5) normal (0, 0, 1) x (1, 0, 0) in component "cassette_2 | Top cassette | DEPTH PROVISIONAL"
sketch "rear_rib_PHOTO_ESTIMATE profile (3)" plane through (0, 0, -177.5) normal (0, 0, 1) x (1, 0, 0) in component "cassette_2 | Top cassette | DEPTH PROVISIONAL"
  line L0 (168.5, 444) -> (175.5, 444)
  line L1 (175.5, 444) -> (175.5, 566)
  line L2 (175.5, 566) -> (168.5, 566)
  line L3 (168.5, 566) -> (168.5, 444)
  line L4 (201.5, 444) -> (208.5, 444)
  line L5 (208.5, 444) -> (208.5, 566)
  line L6 (208.5, 566) -> (201.5, 566)
  line L7 (201.5, 566) -> (201.5, 444)
  line L8 (234.5, 444) -> (241.5, 444)
  line L9 (241.5, 444) -> (241.5, 566)
  line L10 (241.5, 566) -> (234.5, 566)
  line L11 (234.5, 566) -> (234.5, 444)
extrude "rear_rib_PHOTO_ESTIMATE solid extrusion''" add sketch "rear_rib_PHOTO_ESTIMATE profile (3)" along normal blind 4 separate body makes body 153 at (170.8333, 525.3333, -177.5) makes body 154 at (203.8333, 525.3333, -177.5) makes body 155 at (236.8333, 525.3333, -177.5) in component "cassette_2 | Top cassette | DEPTH PROVISIONAL"
ref_plane "WorkPlane5" through (0, 0, -234) normal (0, 0, 1) x (1, 0, 0) in component "cassette_2 | Top cassette | DEPTH PROVISIONAL"
sketch "magnetic_base profile (3)" plane through (0, 0, -234) normal (0, 0, 1) x (1, 0, 0) in component "cassette_2 | Top cassette | DEPTH PROVISIONAL"
  line L0 (191, 436.5) -> (219, 436.5)
  line L1 (219, 436.5) -> (219, 439.5)
  line L2 (219, 439.5) -> (191, 439.5)
  line L3 (191, 439.5) -> (191, 436.5)
extrude "magnetic_base solid extrusion''" add sketch "magnetic_base profile (3)" along normal blind 25 separate body makes body 156 in component "cassette_2 | Top cassette | DEPTH PROVISIONAL"
ref_plane "WorkPlane6" through (0, 0, -269.5) normal (0, 0, 1) x (1, 0, 0) in component "cassette_2 | Top cassette | DEPTH PROVISIONAL"
sketch "center_divider profile (3)" plane through (0, 0, -269.5) normal (0, 0, 1) x (1, 0, 0) in component "cassette_2 | Top cassette | DEPTH PROVISIONAL"
  line L0 (203, 444) -> (207, 444)
  line L1 (207, 444) -> (207, 566)
  line L2 (207, 566) -> (203, 566)
  line L3 (203, 566) -> (203, 444)
extrude "center_divider solid extrusion''" add sketch "center_divider profile (3)" along normal blind 96 separate body makes body 157 in component "cassette_2 | Top cassette | DEPTH PROVISIONAL"
ref_plane "WorkPlane7" through (0, 0, -259.5) normal (0, 0, 1) x (1, 0, 0) in component "cassette_2 | Top cassette | DEPTH PROVISIONAL"
sketch "slide_glass profile (3)" plane through (0, 0, -259.5) normal (0, 0, 1) x (1, 0, 0) in component "cassette_2 | Top cassette | DEPTH PROVISIONAL"
  line L0 (175, 553.5) -> (201, 553.5)
  line L1 (201, 553.5) -> (201, 554.5)
  line L2 (201, 554.5) -> (175, 554.5)
  line L3 (175, 554.5) -> (175, 553.5)
  line L4 (175, 543) -> (201, 543)
  line L5 (201, 543) -> (201, 544)
  line L6 (201, 544) -> (175, 544)
  line L7 (175, 544) -> (175, 543)
  line L8 (175, 532.5) -> (201, 532.5)
  line L9 (201, 532.5) -> (201, 533.5)
  line L10 (201, 533.5) -> (175, 533.5)
  line L11 (175, 533.5) -> (175, 532.5)
  line L12 (175, 522) -> (201, 522)
  line L13 (201, 522) -> (201, 523)
  line L14 (201, 523) -> (175, 523)
  line L15 (175, 523) -> (175, 522)
  line L16 (175, 511.5) -> (201, 511.5)
  line L17 (201, 511.5) -> (201, 512.5)
  line L18 (201, 512.5) -> (175, 512.5)
  line L19 (175, 512.5) -> (175, 511.5)
  line L20 (175, 501) -> (201, 501)
  line L21 (201, 501) -> (201, 502)
  line L22 (201, 502) -> (175, 502)
  line L23 (175, 502) -> (175, 501)
  line L24 (175, 490.5) -> (201, 490.5)
  line L25 (201, 490.5) -> (201, 491.5)
  line L26 (201, 491.5) -> (175, 491.5)
  line L27 (175, 491.5) -> (175, 490.5)
  line L28 (175, 480) -> (201, 480)
  line L29 (201, 480) -> (201, 481)
  line L30 (201, 481) -> (175, 481)
  line L31 (175, 481) -> (175, 480)
  line L32 (175, 469.5) -> (201, 469.5)
  line L33 (201, 469.5) -> (201, 470.5)
  line L34 (201, 470.5) -> (175, 470.5)
  line L35 (175, 470.5) -> (175, 469.5)
  line L36 (175, 459) -> (201, 459)
  line L37 (201, 459) -> (201, 460)
  line L38 (201, 460) -> (175, 460)
  line L39 (175, 460) -> (175, 459)
  line L40 (209, 553.5) -> (235, 553.5)
  line L41 (235, 553.5) -> (235, 554.5)
  line L42 (235, 554.5) -> (209, 554.5)
  line L43 (209, 554.5) -> (209, 553.5)
  line L44 (209, 543) -> (235, 543)
  line L45 (235, 543) -> (235, 544)
  line L46 (235, 544) -> (209, 544)
  line L47 (209, 544) -> (209, 543)
  line L48 (209, 532.5) -> (235, 532.5)
  line L49 (235, 532.5) -> (235, 533.5)
  line L50 (235, 533.5) -> (209, 533.5)
  line L51 (209, 533.5) -> (209, 532.5)
  line L52 (209, 522) -> (235, 522)
  line L53 (235, 522) -> (235, 523)
  line L54 (235, 523) -> (209, 523)
  line L55 (209, 523) -> (209, 522)
  line L56 (209, 511.5) -> (235, 511.5)
  line L57 (235, 511.5) -> (235, 512.5)
  line L58 (235, 512.5) -> (209, 512.5)
  line L59 (209, 512.5) -> (209, 511.5)
  line L60 (209, 501) -> (235, 501)
  line L61 (235, 501) -> (235, 502)
  line L62 (235, 502) -> (209, 502)
  line L63 (209, 502) -> (209, 501)
  line L64 (209, 490.5) -> (235, 490.5)
  line L65 (235, 490.5) -> (235, 491.5)
  line L66 (235, 491.5) -> (209, 491.5)
  line L67 (209, 491.5) -> (209, 490.5)
  line L68 (209, 480) -> (235, 480)
  line L69 (235, 480) -> (235, 481)
  line L70 (235, 481) -> (209, 481)
  line L71 (209, 481) -> (209, 480)
  line L72 (209, 469.5) -> (235, 469.5)
  line L73 (235, 469.5) -> (235, 470.5)
  line L74 (235, 470.5) -> (209, 470.5)
  line L75 (209, 470.5) -> (209, 469.5)
  line L76 (209, 459) -> (235, 459)
  line L77 (235, 459) -> (235, 460)
  line L78 (235, 460) -> (209, 460)
  line L79 (209, 460) -> (209, 459)
extrude "slide_glass solid extrusion''" add sketch "slide_glass profile (3)" along normal blind 76 separate body makes body 158 at (226.3333, 470.5, -234.1667) makes body 159 at (226.3333, 491.5, -234.1667) makes body 160 at (226.3333, 512.5, -234.1667) makes body 161 at (226.3333, 533.5, -234.1667) makes body 162 at (226.3333, 554.5, -234.1667) makes body 163 at (192.3333, 460, -234.1667) makes body 164 at (192.3333, 481, -234.1667) makes body 165 at (192.3333, 502, -234.1667) makes body 166 at (192.3333, 523, -234.1667) makes body 167 at (192.3333, 544, -234.1667) makes body 168 at (192.3333, 533.5, -234.1667) makes body 169 at (192.3333, 512.5, -234.1667) makes body 170 at (192.3333, 491.5, -234.1667) makes body 171 at (192.3333, 470.5, -234.1667) makes body 172 at (192.3333, 554.5, -234.1667) makes body 173 at (226.3333, 544, -234.1667) makes body 174 at (226.3333, 523, -234.1667) makes body 175 at (226.3333, 502, -234.1667) makes body 176 at (226.3333, 481, -234.1667) makes body 177 at (226.3333, 460, -234.1667) in component "cassette_2 | Top cassette | DEPTH PROVISIONAL"
ref_plane "WorkPlane8" through (0, 0, -263) normal (0, 0, 1) x (1, 0, 0) in component "cassette_2 | Top cassette | DEPTH PROVISIONAL"